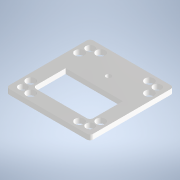
# Autodesk Inventor part: 30_Cube_Z_Focus_MGN_NEMA_counterplate
Saved by Autodesk Inventor 2022 (Build 260153000, 153)
## iProperties
Created: 2017-06-20
Part Number: 30_Cube_Z_Focus_MGN_NEMA_counterplate
Material: Generisch
Document SubType Name: Modeling
Designer: diederichbenedict
Density: 1 g/cm^3
Appearance: Weiß
Mass: 7.87446 g
Surface Area: 71.4468 cm^2
Volume: 7.87446 cm^3
d_part: 50,000 mm
d_o: 40,000 mm
d_i: 40,000 mm
Author: diederichbenedict
Autodesk Inventor part; units mm, degrees
ref_plane "YZ Plane" through (0, 0, 0) normal (1, 0, 0) x (0, 1, 0)
ref_plane "XZ Plane" through (0, 0, 0) normal (0, 1, 0) x (-1, 0, 0)
ref_plane "XY Plane" through (0, 0, 0) normal (0, 0, 1) x (1, 0, 0)
sketch "Skizze1" plane through (0, 0, 0) normal (0, 0, 1) x (1, 0, 0)
  line L0 (-17.4, -0.2) -> (-25.4, -0.2)
  line L1 (-25.4, -0.2) -> (-25.4, -23.2)
  line L2 (-23.4, -25.2) -> (-0.4, -25.2)
  line L3 (-0.4, -25.2) -> (-0.4, -17.2)
  line L4 (-17.4, -0.2) -> (-17.4, -15.2)
  line L5 (-15.4, -17.2) -> (-0.4, -17.2)
  arc A0 (-25.4, -23.2) -> (-23.4, -25.2) centre (-23.4, -23.2) ccw
  circle A1 centre (-20.4, -20.2) radius 2.425
  circle A2 centre (-21.2, -14.7) radius 2.65
  circle A3 centre (-14.9, -21) radius 2.65
  arc A4 (-17.4, -15.2) -> (-15.4, -17.2) centre (-15.4, -15.2) ccw
  circle A5 centre (-20.4, -20.2) radius 2.425
  circle A6 centre (-14.9, -21) radius 2.65
  circle A7 centre (-21.2, -14.7) radius 2.65
  point P0 (-25.4, -25.2)
  point P1 (-17.4, -17.2)
  dimension "d278" = 25
  dimension "d279" = 25
  dimension "d2" = 8
  dimension "d281" = 8
  dimension "d282" = 2
  dimension "d283" = 4.85
  dimension "d284" = 20
  dimension "d4" = 20
  dimension "d286" = 5.3
  dimension "d_hole" = 5.3
  dimension "d290" = 20.8
  dimension "d" = 20.8
  dimension "d292" = 2
  dimension "d313" = 6.3
  dimension "d314" = 6.3
  dimension "d330" = 0
  dimension "d331" = 0
  dimension "d332" = 0
  constraints: 12 end point, 8 centre point, 4 point on circle, 4 point on line, 4 tangent, 2 coincident, 2 parallel, 1 horizontal, 1 perpendicular
  measures "d278" distance of L2.end point (-25.4, -25.2)
  measures "d279" distance of point (-25.4, -25.2) L0.end
  measures "d2" distance between parallel lines of L4 L1
  measures "d281" distance between parallel lines of L2 L5
  measures "d282" radius of A0
  measures "d283" diameter of A1
  measures "d284" distance from line of L0 A1.centre
  measures "d4" distance from line of L3 A1.centre
  measures "d286" diameter of A2
  measures "d_hole" diameter of A3
  measures "d290" distance from line of L0 A3.centre
  measures "d" distance from line of L3 A2.centre
  measures "d292" radius of A4
  measures "d313" horizontal distance of A2.centre A3.centre
  measures "d314" horizontal distance of A2.centre A3.centre
  measures "d330" radial gap between concentric circles of A1 A5
  measures "d331" radial gap between concentric circles of A3 A6
  measures "d332" radial gap between concentric circles of A2 A7
extrude "Extrusion1" add sketch "Skizze1" along normal blind 3
mirror "Mirror6" about plane through (-17.4, -0.2, 0) normal (0, 1, 0) of "Extrusion1"
mirror "Mirror7" about plane through (-0.4, -25.2, 0) normal (1, 0, 0) of "Extrusion1", "Mirror6"
sketch "Sketch32" plane through (0, 0, 3) normal (0, 0, 1) x (1, 0, 0)
  circle A0 centre (-0.54, 11.03) radius 1.4 projected
  circle A1 centre (-0.54, 11.03) radius 7 construction
  circle A2 centre (-0.54, 11.03) radius 1.75 projected
  line L0 (22.6, 24.8) -> (-23.4, 24.8) projected
  arc A3 (-23.4, 24.8) -> (-25.4, 22.8) centre (-23.4, 22.8) ccw projected
  line L1 (-25.4, -23.2) -> (-25.4, 22.8) projected
  arc A4 (-25.4, -23.2) -> (-23.4, -25.2) centre (-23.4, -23.2) ccw projected
  line L2 (-23.4, -25.2) -> (22.6, -25.2) projected
  arc A5 (22.6, -25.2) -> (24.6, -23.2) centre (22.6, -23.2) ccw projected
  line L3 (24.6, 22.8) -> (24.6, -23.2) projected
  arc A6 (24.6, 22.8) -> (22.6, 24.8) centre (22.6, 22.8) ccw projected
  circle A7 centre (19.6, 19.8) radius 2.425 projected
  circle A8 centre (14.1, 20.6) radius 2.65 projected
  circle A9 centre (20.4, 14.3) radius 2.65 projected
  circle A10 centre (19.6, -20.2) radius 2.425 projected
  circle A11 centre (14.1, -21) radius 2.65 projected
  circle A12 centre (20.4, -14.7) radius 2.65 projected
  circle A13 centre (-20.4, 19.8) radius 2.425 projected
  circle A14 centre (-14.9, 20.6) radius 2.65 projected
  circle A15 centre (-21.2, 14.3) radius 2.65 projected
  circle A16 centre (-21.2, -14.7) radius 2.65 projected
  circle A17 centre (-14.9, -21) radius 2.65 projected
  circle A18 centre (-20.4, -20.2) radius 2.425 projected
  line L4 (14.6, 16.8) -> (-15.4, 16.8) projected
  arc A19 (16.6, 14.8) -> (14.6, 16.8) centre (14.6, 14.8) ccw projected
  line L5 (16.6, 14.8) -> (16.6, -15.2) projected
  arc A20 (14.6, -17.2) -> (16.6, -15.2) centre (14.6, -15.2) ccw projected
  line L6 (-15.4, -17.2) -> (14.6, -17.2) projected
  arc A21 (-17.4, -15.2) -> (-15.4, -17.2) centre (-15.4, -15.2) ccw projected
  line L7 (-17.4, -15.2) -> (-17.4, 14.8) projected
  arc A22 (-15.4, 16.8) -> (-17.4, 14.8) centre (-15.4, 14.8) ccw projected
  line L8 (16.6, 14.8) -> (16.6, -15.2) projected
  circle A23 centre (-0.54, 11.03) radius 1.5
  line L9 (16.6, 2.2667) -> (-17.4, 2.2667)
  line L10 (-17.4, -15.2) -> (-17.4, 14.8) projected
  point P0 (0, 0)
  dimension "d354" = 3
  constraints: 2 end point, 2 point on line, 1 centre point, 1 coincident, 1 perpendicular
  measures "d354" diameter of A23
extrude "Extrusion17" add sketch "Sketch32" against normal blind 3 contours A2 | A19 L5 L9 L7 A22 L4
equation "\"d_i\" = 40"
equation "\"d_o\" = 40"
equation "\"d_part\" = 50"
equation "\"d6\" = 0"
equation "\"d7\" = 0"
equation "\"d8\" = 0"
equation "\"d9\" = 0"
equation "\"d13\" = 0"
equation "\"d14\" = 0"
equation "\"d20\" = 0"
equation "\"d21\" = 0"
equation "\"d22\" = 0"
equation "\"d23\" = 0"
equation "\"d24\" = 0"
equation "\"d25\" = 3"
equation "\"d26\" = 0"
equation "\"d27\" = 0"
equation "\"d28\" = 0"
equation "\"d29\" = 0"
equation "\"d30\" = 0"
equation "\"d31\" = 0"
equation "\"d32\" = 0"
equation "\"d33\" = 0"
equation "\"d34\" = 0"
equation "\"d46\" = 0"
equation "\"d47\" = 0"
equation "\"d48\" = 0"
equation "\"d50\" = 0"
equation "\"d51\" = 0"
equation "\"d52\" = 0"
equation "\"d53\" = 0"
equation "\"d54\" = 0"
equation "\"d55\" = 0"
equation "\"d56\" = 0"
equation "\"d57\" = 0"
equation "\"d58\" = 0"
equation "\"d59\" = 0"
equation "\"magnet_offset\" = 0"
equation "\"screw_offset\" = 0"
equation "\"mal_puzzle_offset\" = 0"
equation "\"fem_puzzle_offset\" = 0"
